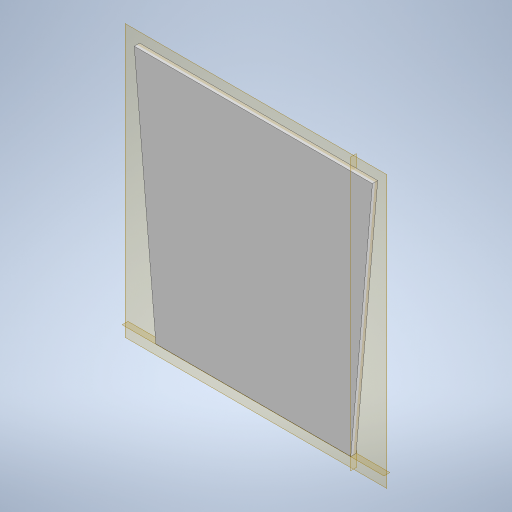
# Autodesk Inventor part: trennwand
Saved by Autodesk Inventor 2023 (Build 270158000, 158)
## iProperties
Created: 2025-07-28
Part Number: trennwand
Material: Generisch
Document SubType Name: Modeling
Designer: johan
Density: 1 g/cm^3
Appearance: Vorgabe
Author: johan
Autodesk Inventor part; units mm, degrees
sketch "Skizze1" plane through (0, 0, 0) normal (0, 0, 1) x (1, 0, 0)
  line L0 (0, 0) -> (-110, 0)
  line L1 (0, 0) -> (12.2018, 139.4673)
  line L2 (0, 0) -> (140, 0) construction
  line L3 (-110, 0) -> (-122.2018, 139.4673)
  line L4 (-110, 0) -> (30, 0) construction
  line L5 (-122.2018, 139.4673) -> (12.2018, 139.4673)
  dimension "d0" = 110
  dimension "d1" = 140
  dimension "d2" = 85
  dimension "d5" = 140
  dimension "d6" = 95
  constraints: 12 end point, 3 horizontal, 2 equal length
  measures "d0" distance of L0.start L0.end
  measures "d1" distance of L0.start L1.end
  measures "d2" angle of L2 L1
  measures "d5" distance of L0.end L3.end
  measures "d6" angle of L4 L3
extrude "Extrusion1" add sketch "Skizze1" along normal mid plane 3
